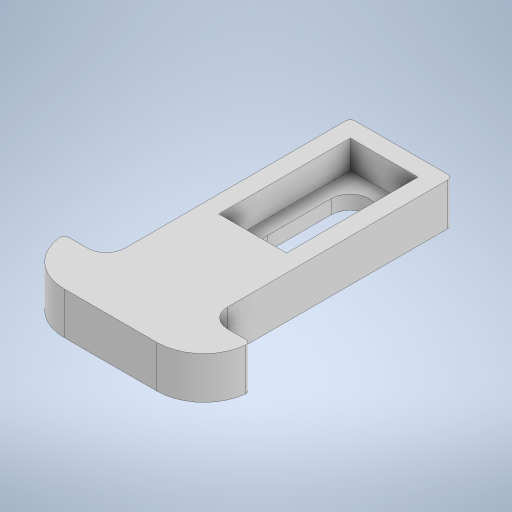
# Autodesk Inventor part: Cierre ventanas
Saved by Autodesk Inventor 2024 (Build 280153000, 153)
## iProperties
Created: 2023-08-26
Part Number: Cierre ventanas
Material: Genérico
Document SubType Name: Modeling
Designer: sergi
Density: 1 g/cm^3
Appearance: Valor por defecto
Author: sergi
Autodesk Inventor part; units mm, degrees
ref_plane "YZ Plane" through (0, 0, 0) normal (1, 0, 0) x (0, 1, 0)
ref_plane "XZ Plane" through (0, 0, 0) normal (0, 1, 0) x (-1, 0, 0)
ref_plane "XY Plane" through (0, 0, 0) normal (0, 0, 1) x (1, 0, 0)
sketch "Boceto1" plane through (0, 0, 0) normal (0, 1, 0) x (-1, 0, 0)
  line L0 (0, 0) -> (10.9, 0)
  line L1 (10.9, 0) -> (10.9, 24)
  line L2 (10.9, 31) -> (0, 31)
  line L3 (0, 24) -> (0, 0)
  line L4 (10.9, 31) -> (10.4, 31)
  line L5 (15.4, 26) -> (15.4, 26)
  line L6 (15.4, 26) -> (12.9, 26)
  line L7 (10.9, 26) -> (10.9, 31)
  line L8 (0, 31) -> (0.5, 31)
  line L9 (-4.5, 26) -> (-4.5, 26)
  line L10 (-4.5, 26) -> (-2, 26)
  line L11 (0, 26) -> (0, 31)
  arc A0 (15.4, 26) -> (10.4, 31) centre (10.4, 26) ccw
  arc A1 (0.5, 31) -> (-4.5, 26) centre (0.5, 26) ccw
  arc A2 (12.9, 26) -> (10.9, 24) centre (12.9, 24) ccw
  arc A3 (0, 24) -> (-2, 26) centre (-2, 24) ccw
  point P0 (15.4, 31)
  point P1 (-4.5, 31)
  dimension "d0" = 10.9
  dimension "d1" = 31
  dimension "d2" = 4.5
  dimension "d3" = 5
  dimension "d4" = 4.5
  dimension "d5" = 5
  dimension "d7" = 5
  dimension "d8" = 5
  dimension "d9" = 2
  constraints: 24 end point, 8 point on circle, 8 point on line, 8 tangent, 6 parallel, 4 centre point, 3 horizontal, 3 perpendicular, 1 equal radius
  measures "d0" distance of L2.end L2.start
  measures "d1" distance of L2.start L0.end
  measures "d2" distance of L5.end L7.start
  measures "d3" distance of point (15.4, 31) L5.end
  measures "d4" distance of L11.start L9.end
  measures "d5" distance of L9.end point (-4.5, 31)
  measures "d7" radius of A0
  measures "d8" radius of A1
  measures "d9" radius of A2
extrude "Extrusión1" add sketch "Boceto1" along normal blind 4.5 contours L3 A3 L10 A1 L2 A0 L6 A2 L1 L0
sketch "Boceto2" plane through (0, 4.5, 0) normal (0, 1, 0) x (1, 0, 0)
  arc A0 (-15.4, -26) -> (-10.4, -31) centre (-10.4, -26) ccw projected
  line L0 (-10.4, -31) -> (-0.5, -31) projected
  arc A1 (-0.5, -31) -> (4.5, -26) centre (-0.5, -26) ccw projected
  line L1 (4.5, -26) -> (2, -26) projected
  arc A2 (0, -24) -> (2, -26) centre (2, -24) ccw projected
  line L2 (0, -24) -> (0, 0) projected
  line L3 (0, 0) -> (-10.9, 0) projected
  line L4 (-10.9, 0) -> (-10.9, -24) projected
  arc A3 (-12.9, -26) -> (-10.9, -24) centre (-12.9, -24) ccw projected
  line L5 (-12.9, -26) -> (-15.4, -26) projected
  line L6 (-9.05, -24) -> (-9.05, -1.85)
  line L7 (-9.05, -1.85) -> (-1.85, -1.85)
  line L8 (-1.85, -1.85) -> (-1.85, -24)
  arc A4 (-1.85, -24) -> (2, -27.85) centre (2, -24) ccw
  line L9 (2, -27.85) -> (2.0495, -27.85)
  arc A5 (-0.5, -29.15) -> (2.0495, -27.85) centre (-0.5, -26) ccw
  line L10 (-0.5, -29.15) -> (-10.4, -29.15)
  arc A6 (-12.9495, -27.85) -> (-10.4, -29.15) centre (-10.4, -26) ccw
  line L11 (-12.9495, -27.85) -> (-12.9, -27.85)
  arc A7 (-12.9, -27.85) -> (-9.05, -24) centre (-12.9, -24) ccw
  line L12 (-5.45, -1.85) -> (-5.45, -15.85)
  line L13 (-5.45, -15.85) -> (-9.05, -15.85)
  line L14 (-5.45, -15.85) -> (-1.85, -15.85)
  dimension "d14" = 7.2
  dimension "d15" = 14
  constraints: 18 end point, 8 point on circle, 4 centre point, 3 point on line, 1 horizontal, 1 midpoint, 1 vertical, 9 other
  measures "d14" distance between parallel lines of L8 L6
  measures "d15" distance of L12.start L12.end
extrude "Extrusión2" cut sketch "Boceto2" against normal blind 3 contours L6 L7 L12 L13 | L12 L7 L8 L14
sketch "Boceto3" plane through (0, 1.5, 0) normal (0, 1, 0) x (1, 0, 0)
  line L0 (-1.85, -1.85) -> (-1.85, -15.85) projected
  line L1 (-9.05, -1.85) -> (-1.85, -1.85) projected
  line L2 (-9.05, -15.85) -> (-9.05, -1.85) projected
  line L3 (-1.85, -15.85) -> (-9.05, -15.85) projected
  line L4 (-5.45, -3.4) -> (-5.45, -3.4)
  line L5 (-3.4, -5.45) -> (-3.4, -12.25)
  line L6 (-5.45, -14.3) -> (-5.45, -14.3)
  line L7 (-7.5, -12.25) -> (-7.5, -5.45)
  arc A0 (-5.45, -3.4) -> (-7.5, -5.45) centre (-5.45, -5.45) ccw
  arc A1 (-5.45, -14.3) -> (-3.4, -12.25) centre (-5.45, -12.25) ccw
  arc A2 (-7.5, -12.25) -> (-5.45, -14.3) centre (-5.45, -12.25) ccw
  arc A3 (-3.4, -5.45) -> (-5.45, -3.4) centre (-5.45, -5.45) ccw
  point P0 (0, 0)
  dimension "d18" = 4.1
  dimension "d19" = 2.05
  constraints: 8 end point, 8 point on circle, 8 tangent, 4 centre point, 3 equal radius, 3 other
  measures "d18" distance between parallel lines of L5 L7
  measures "d19" radius of A0
extrude "Extrusión3" cut sketch "Boceto3" against normal blind 3 contours L5 A1 A2 L7 A0 A3
fillet "Empalme1" radius 0.5 4 edges at (0, 2.25, 0) (-10.9, 2.25, 0) (4.5, 2.25, 26) (-15.4, 2.25, 26)
